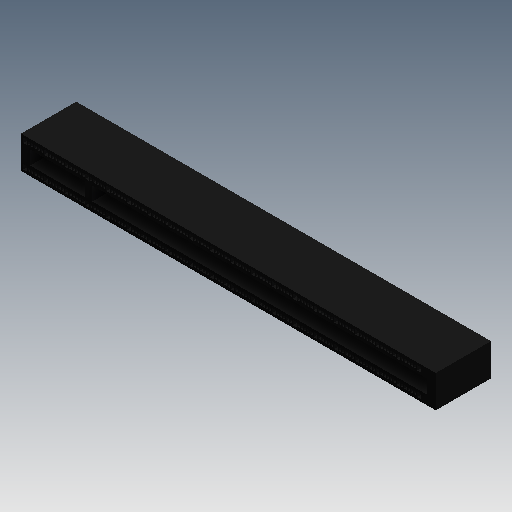
# Autodesk Inventor part: config - agp slot
Saved by Autodesk Inventor 2019.1 (Build 231200000, 200)
## iProperties
Company: Autodesk Asia Pte. Ltd.
Created: 2005-12-05
Part Number: config - agp slot
Document SubType Name: Modeling
Designer: Simon.Ng@autodesk.com
Stock Number: config - agp slot
Density: 1 g/cm^3
Material: Generic
Mass: 5.0822 g
Surface Area: 78.676 cm^2
Volume: 5.0822 cm^3
Appearance: Glossy - Black
Title: PC Demo
Author: Simon.Ng@autodesk.com
Autodesk Inventor part; units mm, degrees
ref_plane "YZ Plane" through (0, 0, 0) normal (1, 0, 0) x (0, 1, 0)
ref_plane "XZ Plane" through (0, 0, 0) normal (0, 1, 0) x (-1, 0, 0)
ref_plane "XY Plane" through (0, 0, 0) normal (0, 0, 1) x (1, 0, 0)
sketch "Sketch1" plane through (0, 0, 0) normal (0, 0, 1) x (1, 0, 0)
  line L0 (0, 5.6) -> (0, -4.2) construction
  line L1 (-54, 0) -> (72, 0) construction
  line L2 (-45, 3.5) -> (45, 3.5)
  line L3 (45, 3.5) -> (45, -3.5)
  line L4 (45, -3.5) -> (-45, -3.5)
  line L5 (-45, -3.5) -> (-45, 3.5)
  dimension "d0" = 90
  dimension "d1" = 7
  constraints: 8 end point, 2 parallel, 1 horizontal, 1 perpendicular, 2 other
  measures "d0" distance of L2.start L2.end
  measures "d1" distance of L4.end L2.start
extrude "Extrusion1" add sketch "Sketch1" along normal blind 12
sketch "Sketch2" plane through (0, 0, 12) normal (0, 0, 1) x (1, 0, 0)
  line L0 (45, 3.5) -> (45, -3.5) projected
  line L1 (-45, -3.5) -> (-45, 3.5) projected
  line L2 (-45, 0) -> (45, 0) construction
  line L3 (-43, 1.5) -> (-31, 1.5)
  line L4 (-31, 1.5) -> (-31, -1.5)
  line L5 (-31, -1.5) -> (-43, -1.5)
  line L6 (-43, -1.5) -> (-43, 1.5)
  line L7 (-29.5, 1.5) -> (43, 1.5)
  line L8 (43, 1.5) -> (43, -1.5)
  line L9 (43, -1.5) -> (-29.5, -1.5)
  line L10 (-29.5, -1.5) -> (-29.5, 1.5)
  dimension "d4" = 2
  dimension "d5" = 3
  dimension "d6" = 12
  dimension "d7" = 1.5
  dimension "d8" = 2
  dimension "d9" = 72.5
  constraints: 18 end point, 4 parallel, 2 horizontal, 2 midpoint, 2 perpendicular, 1 collinear, 2 other
  measures "d4" distance between parallel lines of L1 L6
  measures "d5" distance of L5.end L3.start
  measures "d6" distance of L3.start L3.end
  measures "d7" distance between parallel lines of L10 L4
  measures "d8" distance between parallel lines of L0 L8
  measures "d9" distance of L7.start L7.end
extrude "Extrusion2" cut sketch "Sketch2" against normal blind 8
sketch "Sketch3" plane through (0, 0, 12) normal (0, 0, 1) x (1, 0, 0)
  line L0 (-43, 1.5) -> (-31, 1.5) projected
  line L1 (-45, 3.5) -> (45, 3.5) projected
  line L2 (-45, -3.5) -> (-45, 3.5) projected
  line L3 (-27.2504, 3.5) -> (-27.2504, 1.5) construction
  line L4 (-27.2504, 2.5) -> (-45, 2.5) construction
  line L5 (-44.5, 3) -> (-43.7, 3)
  line L6 (-43.7, 3) -> (-43.7, 2)
  line L7 (-43.7, 2) -> (-44.5, 2)
  line L8 (-44.5, 2) -> (-44.5, 3)
  line L9 (-43.5, 2.8) -> (-43, 2.8)
  line L10 (-43, 2.8) -> (-43, 2.2)
  line L11 (-43, 2.2) -> (-43.5, 2.2)
  line L12 (-43.5, 2.2) -> (-43.5, 2.8)
  line L13 (-42.8, 2.8) -> (-42.3, 2.8)
  line L14 (-42.3, 2.8) -> (-42.3, 2.2)
  line L15 (-42.3, 2.2) -> (-42.8, 2.2)
  line L16 (-42.8, 2.2) -> (-42.8, 2.8)
  line L17 (-42.1, 2.8) -> (-41.6, 2.8)
  line L18 (-41.6, 2.8) -> (-41.6, 2.2)
  line L19 (-41.6, 2.2) -> (-42.1, 2.2)
  line L20 (-42.1, 2.2) -> (-42.1, 2.8)
  line L21 (-41.4, 2.8) -> (-40.9, 2.8)
  line L22 (-40.9, 2.8) -> (-40.9, 2.2)
  line L23 (-40.9, 2.2) -> (-41.4, 2.2)
  line L24 (-41.4, 2.2) -> (-41.4, 2.8)
  line L25 (-40.7, 2.8) -> (-40.2, 2.8)
  line L26 (-40.2, 2.8) -> (-40.2, 2.2)
  line L27 (-40.2, 2.2) -> (-40.7, 2.2)
  line L28 (-40.7, 2.2) -> (-40.7, 2.8)
  dimension "d12" = 0.8
  dimension "d13" = 1
  dimension "d14" = 0.2
  dimension "d15" = 0.5
  dimension "d16" = 0.5
  dimension "d17" = 0.6
  dimension "d20" = 0.7
  constraints: 52 end point, 4 parallel, 4 perpendicular, 3 horizontal, 3 point on line, 1 midpoint, 34 other
  measures "d12" distance of L5.start L5.end
  measures "d13" distance of L7.end L5.start
  measures "d14" distance between parallel lines of L6 L12
  measures "d15" distance between parallel lines of L2 L8
  measures "d16" distance of L9.start L9.end
  measures "d17" distance of L9.end L10.end
  measures "d20" distance of L9.start L13.start
extrude "Extrusion3" cut sketch "Sketch3" against normal blind 5
pattern_linear "Rectangular Pattern1" count 19 spacing 4.5 along (1, 0, 0) count 2 spacing 5 along (0, -1, 0) of "Extrusion3"
sketch "Sketch4" plane through (0, 0, 12) normal (0, 0, 1) x (1, 0, 0)
  line L0 (18.5, -2) -> (19.3, -2) projected
  line L1 (19.3, -3) -> (18.5, -3) projected
  line L2 (27.5, 3) -> (28.3, 3) projected
  line L3 (28.3, 2) -> (27.5, 2) projected
  line L4 (41, 3) -> (41.8, 3)
  line L5 (41.8, 3) -> (41.8, 2)
  line L6 (41.8, 2) -> (41, 2)
  line L7 (41, 2) -> (41, 3)
  line L8 (41, -2) -> (41.8, -2)
  line L9 (41.8, -2) -> (41.8, -3)
  line L10 (41.8, -3) -> (41, -3)
  line L11 (41, -3) -> (41, -2)
  line L12 (40.8, -2.2) -> (40.8, -2.8) projected
  dimension "d34" = 0.8
  dimension "d38" = 0.2
  constraints: 16 end point, 6 collinear, 4 parallel, 2 horizontal, 2 perpendicular
  measures "d34" distance of L9.end L10.end
  measures "d38" distance between parallel lines of L12 L11
extrude "Extrusion4" cut sketch "Sketch4" against normal blind 8
body "Solid1"
